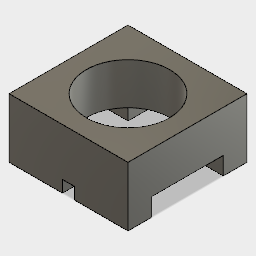
soporte motor (Autodesk Fusion 360 design; units mm, degrees)
Autodesk Fusion 360 part; units mm, degrees
sketch "Sketch1" plane through (0, 0, 0) normal (0, 1, 0) x (1, 0, 0)
  line L0 (20, 20) -> (-20, 20)
  line L1 (-20, 20) -> (-20, -20)
  line L2 (-20, -20) -> (20, -20)
  line L3 (20, -20) -> (20, 20)
  line L4 (20, 20) -> (-20, -20) construction
  line L5 (-20, 20) -> (20, -20) construction
  dimension "d1" = 40
  measures "d1" distance of L1.end L2.end
extrude "Extrude1" add sketch "Sketch1" along normal blind 20
sketch "Sketch2" plane through (0, 20, 0) normal (0, 1, 0) x (-1, 0, 0)
  line L0 (-20, 20) -> (-20, -20)
  line L1 (-20, -20) -> (20, -20)
  line L2 (20, -20) -> (20, 20)
  line L3 (20, 20) -> (-20, 20)
hole "Hole1" at (0, 20, 0) direction (0, -1, 0) diameter 28 end through all
sketch "Sketch3" plane through (0, 0, 20) normal (0, 0, 1) x (1, 0, 0)
  line L0 (-20, 0) -> (20, 0)
  line L1 (20, 0) -> (20, 20)
  line L2 (20, 20) -> (-20, 20)
  line L3 (-20, 20) -> (-20, 0)
  line L4 (2, 4) -> (-2, 4)
  line L5 (-2, 4) -> (-2, -4)
  line L6 (-2, -4) -> (2, -4)
  line L7 (2, -4) -> (2, 4)
  line L8 (2, 4) -> (-2, -4) construction
  line L9 (-2, 4) -> (2, -4) construction
  dimension "d7" = 4
  dimension "d8" = 8
  measures "d7" distance of L5.end L6.end
  measures "d8" distance of L4.end L5.end
extrude "Extrude2" cut sketch "Sketch3" against normal blind 10 contours L0 L4 L5 L7
sketch "Sketch4" plane through (0, 0, 0) normal (0, -1, 0) x (1, 0, 0)
  line L0 (-2, 13.8564) -> (-2, 20)
  line L1 (-2, 20) -> (-20, 20)
  line L2 (-20, 20) -> (-20, -20)
  line L3 (-20, -20) -> (20, -20)
  line L4 (20, -20) -> (20, 20)
  line L5 (20, 20) -> (2, 20)
  line L6 (2, 20) -> (2, 13.8564)
  arc A0 (-2, 13.8564) -> (2, 13.8564) centre (0, 0) ccw
  line L7 (25, -12) -> (5, -12)
  line L8 (5, -12) -> (5, 12)
  line L9 (5, 12) -> (25, 12)
  line L10 (25, 12) -> (25, -12)
  line L11 (25, -12) -> (5, 12) construction
  line L12 (5, -12) -> (25, 12) construction
  point P0 (15, 0)
extrude "Extrude3" cut sketch "Sketch4" against normal blind 6 contours L4 A0 L7 L9
sketch "Sketch5" plane through (0, 0, 0) normal (0, -1, 0) x (1, 0, 0)
  line L0 (20, -12) -> (7.2111, -12)
  arc A0 (-2, 13.8564) -> (7.2111, -12) centre (0, 0) ccw
  line L1 (-2, 13.8564) -> (-2, 20)
  line L2 (-2, 20) -> (-20, 20)
  line L3 (-20, 20) -> (-20, -20)
  line L4 (-20, -20) -> (20, -20)
  line L5 (20, -20) -> (20, -12)
  line L6 (12, -9) -> (-12, -9)
  line L7 (-12, -9) -> (-12, -31)
  line L8 (-12, -31) -> (12, -31)
  line L9 (12, -31) -> (12, -9)
  line L10 (12, -9) -> (-12, -31) construction
  line L11 (-12, -9) -> (12, -31) construction
  point P0 (0, -20)
extrude "Extrude4" cut sketch "Sketch5" against normal blind 6 contours L0 A0 L4 L6 L7 L9
sketch "Sketch6" plane through (0, 0, 0) normal (0, -1, 0) x (1, 0, 0)
  line L0 (-12, -20) -> (-12, -9)
  line L1 (-12, -9) -> (-10.7238, -9)
  arc A0 (-2, 13.8564) -> (-10.7238, -9) centre (0, 0) ccw
  line L2 (-2, 13.8564) -> (-2, 20)
  line L3 (-2, 20) -> (-20, 20)
  line L4 (-20, 20) -> (-20, -20)
  line L5 (-20, -20) -> (-12, -20)
  line L6 (-4, 12) -> (-36, 12)
  line L7 (-36, 12) -> (-36, -12)
  line L8 (-36, -12) -> (-4, -12)
  line L9 (-4, -12) -> (-4, 12)
  line L10 (-4, 12) -> (-36, -12) construction
  line L11 (-36, 12) -> (-4, -12) construction
  point P0 (-20, 0)
extrude "Extrude5" cut sketch "Sketch6" against normal blind 6 contours L0 L1 A0 L4 L6 L8
